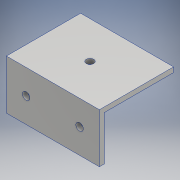
# Autodesk Inventor part: bepf_podwozie_lacznik_glownego_wspornika
Saved by Autodesk Inventor 2017 (Build 210142000, 142)
## iProperties
Created: 2016-11-23
Part Number: bepf_podwozie_lacznik_glownego_wspornika
Material: Aluminium 6061
Document SubType Name: Modeling
Designer: gagato
Density: 2.7 g/cm^3
Appearance: Aluminium — płaski
Mass: 9.63141 g
Surface Area: 39.6614 cm^2
Volume: 3.56719 cm^3
Author: gagato
Autodesk Inventor part; units mm, degrees
ref_plane "YZ Plane" through (0, 0, 0) normal (1, 0, 0) x (0, 1, 0)
ref_plane "XZ Plane" through (0, 0, 0) normal (0, 1, 0) x (-1, 0, 0)
ref_plane "XY Plane" through (0, 0, 0) normal (0, 0, 1) x (1, 0, 0)
sketch "Szkic1" plane through (0, 0, 0) normal (1, 0, 0) x (0, 1, 0)
  line L0 (2, 0) -> (30, 0)
  line L1 (30, 0) -> (30, -2)
  line L2 (30, -2) -> (2, -2)
  line L3 (2, 0) -> (0, 0)
  line L4 (0, 0) -> (0, -20)
  line L5 (0, -20) -> (2, -20)
  line L6 (2, -20) -> (2, -2)
  dimension "d2" = 2
  dimension "d7" = 30
  dimension "d8" = 20
  dimension "d9" = 2
  constraints: 14 end point, 3 parallel, 2 horizontal, 2 perpendicular, 1 coincident, 1 point on line
  measures "d2" distance of L5.end L4.end
  measures "d7" distance of L3.end L0.end
  measures "d8" distance of L3.end L4.end
  measures "d9" distance of L0.end L1.end
extrude "Wyciągnięcie proste1" add sketch "Szkic1" along normal mid plane 37.6
sketch "Szkic2" plane through (-18.8, 0, 0) normal (0, 0, 1) x (1, 0, 0)
  line L0 (18.8, 0) -> (18.8, 15) construction
  dimension "d12" = 15
  constraints: 2 end point, 1 coincident, 1 vertical
  measures "d12" distance of L0.start L0.end
hole "Otwór1" at (0, 15, 0) direction (0, 0, -1) diameter 3 end through all
sketch "Szkic3" plane through (-18.8, 0, -20) normal (0, -1, 0) x (1, 0, 0)
  line L0 (0, 0) -> (0, 20) projected
  line L1 (37.6, 20) -> (37.6, 0) projected
  line L2 (0, 10) -> (8, 10) construction
  line L3 (37.6, 10) -> (29.6, 10) construction
  point P0 (18.8, 20)
  dimension "d20" = 8
  dimension "d21" = 8
  constraints: 4 end point, 2 coincident, 2 horizontal, 2 midpoint
  measures "d20" distance of L2.start L2.end
  measures "d21" distance of L3.start L3.end
hole "Otwór2" at (-10.8, 0, -10) at (10.8, 0, -10) direction (0, 1, 0) diameter 3 end through all
